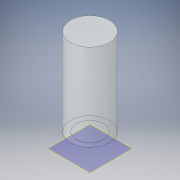
# Autodesk Inventor part: edmunds_20x
Saved by Autodesk Inventor 2017 (Build 210142000, 142)
## iProperties
Created: 2017-03-12
Part Number: edmunds_20x
Material: Glass
Document SubType Name: Modeling
Designer: richp
Density: 2.18 g/cm^3
Appearance: Clear
EO_20x_diameter: 1.339 in
E0_20x_front_aperture_diameter: 0.945 in
Author: richp
Autodesk Inventor part; units mm, degrees
ref_plane "YZ Plane" through (0, 0, 0) normal (1, 0, 0) x (0, 1, 0)
ref_plane "XZ Plane" through (0, 0, 0) normal (0, 1, 0) x (-1, 0, 0)
ref_plane "XY Plane" through (0, 0, 0) normal (0, 0, 1) x (1, 0, 0)
sketch "Sketch1" plane through (0, 0, 0) normal (0, 1, 0) x (-1, 0, 0)
  circle A0 centre (0, 0) radius 17
  dimension "EO_20x_diameter" = 33.9999
  constraints: 1 centre point, 1 coincident
  measures "EO_20x_diameter" diameter of A0
extrude "Extrusion1" add sketch "Sketch1" along normal blind 76.2
ref_plane "Work Plane1" through (0, -13, 0) normal (0, -1, 0) x (1, 0, 0)
sketch "Sketch3" plane through (0, -13, 0) normal (0, -1, 0) x (1, 0, 0)
  circle A0 centre (0, 0) radius 0.22
  dimension "d4" = 0.44
  constraints: 1 centre point, 1 coincident
  measures "d4" diameter of A0
sketch "Sketch4" plane through (0, 0, 0) normal (0, -1, 0) x (1, 0, 0)
  circle A0 centre (0, 0) radius 12
  dimension "E0_20x_front_aperture_diameter" = 24
  constraints: 1 centre point, 1 coincident
  measures "E0_20x_front_aperture_diameter" diameter of A0
loft "Loft2" add profiles "Sketch4", "Sketch3"
body "Solid1"
